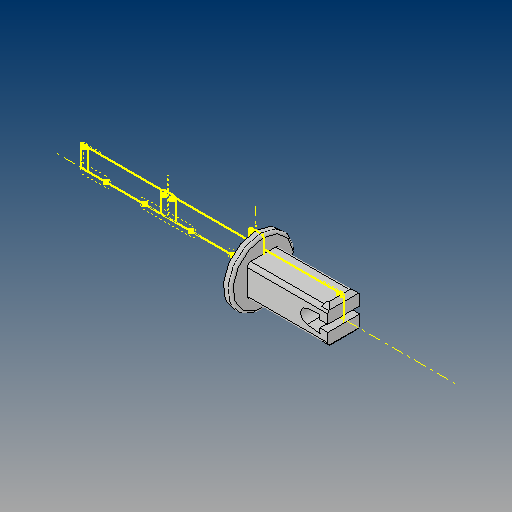
# Autodesk Inventor part: Connector_pin_base
Saved by Autodesk Inventor 2020 (Build 240168000, 168)
## iProperties
Created: 2019-02-01
Part Number: Connector_pin_base
Material: Generic
Document SubType Name: Modeling
Designer: Varga Daniel
Density: 1 g/cm^3
Appearance: Default
Author: Varga Daniel
Autodesk Inventor part; units mm, degrees
ref_plane "YZ Plane" through (0, 0, 0) normal (1, 0, 0) x (0, 1, 0)
ref_plane "XZ Plane" through (0, 0, 0) normal (0, 1, 0) x (-1, 0, 0)
ref_plane "XY Plane" through (0, 0, 0) normal (0, 0, 1) x (1, 0, 0)
derived "Base_part.ipt"
derived "Connector_pin_base.ipt"
sketch "Pin_base_sketch" plane through (0, 0, 0) normal (0, 0, 1) x (1, 0, 0)
  line L0 (0, 0) -> (23.0918, 0) construction
  line L1 (0, 0) -> (0, 6.22) construction
  line L2 (0, 3.75) -> (0.525, 3.75)
  line L3 (0.825, 3.45) -> (0.825, 2.4)
  line L4 (0.825, 2.4) -> (9.225, 2.4)
  line L5 (0, 0) -> (0, 3.75)
  line L6 (0, 0) -> (3.25, 0)
  arc A0 (0.825, 3.45) -> (0.525, 3.75) centre (0.525, 3.45) ccw
  line L7 (0.825, 2.4) -> (0.825, 0.575)
  line L8 (0, 0) -> (-23.0918, 0) construction
  line L9 (9.225, 2.4) -> (9.225, 0.575)
  line L10 (10.025, 2.4) -> (10.025, 2.1865) construction
  line L11 (9.225, 2.4) -> (10.025, 2.4) construction
  line L12 (9.625, 2.4) -> (9.625, 0) construction
  line L13 (10.1291, 2.615) -> (7.4184, 2.615) construction
  line L14 (10.025, 0.575) -> (9.225, 0.575) construction
  line L15 (10.025, 0.575) -> (10.025, 0)
  arc A1 (7.1, 0.575) -> (6.525, 0) centre (7.1, 0) ccw construction
  line L16 (9.225, 0.575) -> (7.1, 0.575) construction
  line L17 (9.225, 0.575) -> (9.225, 0)
  line L18 (0, 0.575) -> (0.825, 0.575) construction
  arc A2 (3.25, 0) -> (2.675, 0.575) centre (2.675, 0) ccw construction
  line L19 (0.825, 0.575) -> (0.825, 0)
  line L20 (0.825, 0.575) -> (2.675, 0.575) construction
  line L21 (0, 0) -> (-3.25, 0)
  line L22 (0, 3.75) -> (-0.525, 3.75)
  line L23 (-0.825, 3.45) -> (-0.825, 2.4)
  arc A3 (-0.525, 3.75) -> (-0.825, 3.45) centre (-0.525, 3.45) ccw
  line L24 (-0.825, 2.4) -> (-0.825, 0.575)
  line L25 (-0.825, 0.575) -> (-0.825, 0)
  line L26 (0, 0.575) -> (-0.825, 0.575) construction
  line L27 (-0.825, 2.4) -> (-9.225, 2.4)
  line L28 (-9.225, 2.4) -> (-9.225, 0)
  line L29 (-10.875, 2.4) -> (-10.875, 0)
  line L30 (-10.5179, 2.55) -> (-9.5821, 2.55)
  line L31 (-10.05, 2.55) -> (-10.05, 0) construction
  line L32 (-9.225, 2.4) -> (-10.875, 2.4) construction
  arc A4 (-10.5179, 2.55) -> (-10.875, 2.4) centre (-10.5179, 2.05) ccw
  arc A5 (-9.225, 2.4) -> (-9.5821, 2.55) centre (-9.5821, 2.05) ccw
  line L33 (-10.875, 2.4) -> (-19.275, 2.4)
  line L34 (-19.275, 2.4) -> (-19.275, 0)
  line L35 (-19.275, 0) -> (-16.575, 0)
  line L36 (-19.275, 2.4) -> (-20.075, 2.4) construction
  line L37 (-20.075, 2.4) -> (-20.075, 2.1865) construction
  line L38 (-20.075, 0) -> (-19.275, 0)
  line L39 (-19.675, 2.4) -> (-19.675, 0) construction
  line L40 (-19.6465, 2.615) -> (-17.4324, 2.615) construction
  line L41 (-0.825, 0.575) -> (-2.675, 0.575) construction
  arc A6 (-2.675, 0.575) -> (-3.25, 0) centre (-2.675, 0) ccw construction
  line L42 (-12.725, 0.575) -> (-7.375, 0.575) construction
  arc A7 (-6.8, 0) -> (-7.375, 0.575) centre (-7.375, 0) ccw construction
  arc A8 (-12.725, 0.575) -> (-13.3, 0) centre (-12.725, 0) ccw construction
  line L43 (-20.075, 0.575) -> (-17.15, 0.575) construction
  arc A9 (-16.575, 0) -> (-17.15, 0.575) centre (-17.15, 0) ccw construction
  line L44 (-16.575, 0) -> (-13.3, 0)
  line L45 (-20.075, 0.575) -> (-20.075, 0)
  line L46 (-13.3, 0) -> (-10.875, 0)
  line L47 (-6.8, 0) -> (-10.875, 0)
  line L48 (-3.25, 0) -> (-6.8, 0)
  line L49 (3.25, 0) -> (6.525, 0)
  line L50 (6.525, 0) -> (10.025, 0)
  arc A10 (-17.15, -0.575) -> (-16.575, 0) centre (-17.15, 0) ccw construction
  line L51 (-20.075, -0.575) -> (-20.075, 0) construction
  line L52 (-20.075, -0.575) -> (-17.15, -0.575) construction
  line L53 (-12.725, -0.575) -> (-7.375, -0.575) construction
  arc A11 (-13.3, 0) -> (-12.725, -0.575) centre (-12.725, 0) ccw construction
  arc A12 (-7.375, -0.575) -> (-6.8, 0) centre (-7.375, 0) ccw construction
  arc A13 (-3.25, 0) -> (-2.675, -0.575) centre (-2.675, 0) ccw construction
  line L54 (-0.825, -0.575) -> (-2.675, -0.575) construction
  line L55 (0, -0.575) -> (-0.825, -0.575) construction
  line L56 (0, -0.575) -> (0.825, -0.575) construction
  line L57 (0.825, -0.575) -> (2.675, -0.575) construction
  arc A14 (2.675, -0.575) -> (3.25, 0) centre (2.675, 0) ccw construction
  arc A15 (6.525, 0) -> (7.1, -0.575) centre (7.1, 0) ccw construction
  line L58 (9.225, -0.575) -> (7.1, -0.575) construction
  line L59 (10.025, -0.575) -> (9.225, -0.575) construction
  line L60 (10.025, -0.575) -> (10.025, 0) construction
  line L61 (-0.025, 0) -> (-0.025, 4.3146) construction
  line L62 (0.025, 0) -> (0.025, 4.3146) construction
  line L63 (-10.075, 0) -> (-10.075, 4.2477) construction
  line L64 (-10.025, 0) -> (-10.025, 4.2339) construction
  arc A16 (-19.275, 2.4) -> (-20.075, 2.1865) centre (-19.6465, 2.1865) ccw
  line L65 (-20.075, 2.1865) -> (-20.075, 0.575)
  arc A17 (10.025, 2.1865) -> (9.225, 2.4) centre (9.5965, 2.1865) ccw
  line L66 (10.025, 2.1865) -> (10.025, 0.575)
sketch "Square_pin_base_sketch" plane through (0, 0, 0) normal (0, 0, 1) x (1, 0, 0)
  line L0 (0, 0) -> (23.0918, 0) construction
  line L1 (0, 3.75) -> (0.525, 3.75)
  line L2 (0.825, 3.45) -> (0.825, 1.825)
  line L3 (0.825, 1.825) -> (9.225, 1.825)
  line L4 (0, 0) -> (0, 3.75)
  line L5 (0, 0) -> (3.25, 0)
  arc A0 (0.825, 3.45) -> (0.525, 3.75) centre (0.525, 3.45) ccw
  line L6 (0.825, 1.825) -> (0.825, 0.575)
  line L7 (0, 0) -> (-23.0918, 0) construction
  line L8 (9.225, 1.825) -> (9.225, 0)
  line L9 (10.025, 1.825) -> (10.025, 1.725) construction
  line L10 (9.225, 1.825) -> (10.025, 1.825) construction
  line L11 (9.625, 2.175) -> (9.625, 0) construction
  line L12 (10.1291, 2.175) -> (7.4184, 2.175) construction
  line L13 (10.025, 0.4) -> (10.025, 0)
  line L14 (0, 0.575) -> (0.825, 0.575)
  arc A1 (3.25, 0) -> (2.675, 0.575) centre (2.675, 0) ccw
  line L15 (0.825, 0.575) -> (0.825, -0.575)
  line L16 (0.825, 0.575) -> (2.675, 0.575)
  line L17 (3.25, 0) -> (6.525, 0)
  line L18 (6.525, 0) -> (10.025, 0)
  line L19 (0, -0.575) -> (0.825, -0.575)
  arc A2 (2.675, -0.575) -> (3.25, 0) centre (2.675, 0) ccw
  line L20 (0.825, -0.575) -> (2.675, -0.575)
  line L21 (10.025, -0.4) -> (10.025, 0) construction
  line L22 (0.025, 0) -> (0.025, 4.3146) construction
  line L23 (10.025, 1.725) -> (10.025, 0)
  line L24 (0, 0.575) -> (0, 0)
  line L25 (0, 0) -> (0, -0.575)
  line L26 (9.625, 2.175) -> (10.025, 1.725)
  arc A3 (9.625, 2.175) -> (9.225, 1.825) centre (9.625, 1.7714) ccw
  line L27 (0, 0) -> (0, 5.1403) construction
  line L28 (10.025, 0.4) -> (9.125, 0.4)
  line L29 (9.125, 0.4) -> (9.125, 0.95)
  line L30 (9.125, 0.95) -> (7.6479, 0.8)
  arc A4 (7.6479, 0.8) -> (6.925, 0) centre (7.7291, 0) ccw
  point P0 (0.825, 0)
  point P1 (-9.225, 0)
  point P2 (-10.875, 0)
  point P3 (-20.075, 0)
  dimension "d237" = 3.65
  dimension "d240" = 0.025
  dimension "d241" = 0.825
  dimension "d242" = 0.3
  dimension "d243" = 7.5
  dimension "d244" = 1.15
  dimension "d245" = 6.5
  dimension "d246" = 8.4
  dimension "d247" = 10
  dimension "d248" = 3.45
  dimension "d249" = 4.35
  dimension "d250" = 0.8
  dimension "d251" = 0.8
  dimension "d252" = 0.9
  dimension "d253" = 1.6
  dimension "d254" = 1.9
  dimension "d255" = 2.3
  constraints: 63 end point, 21 point on line, 13 perpendicular, 10 point on circle, 7 horizontal, 6 tangent, 5 centre point, 4 symmetric about line, 3 collinear, 2 vertical, 1 midpoint, 1 parallel, 3 other
  measures "d237" diameter of L3 L0
  measures "d240" distance between parallel lines of L22 L27
  measures "d241" distance between parallel lines of L4 L2
  measures "d242" radius of A0
  measures "d243" diameter of L1 L7
  measures "d244" distance between parallel lines of L20 L16
  measures "d245" diameter of L5.end L27
  measures "d246" distance between parallel lines of L6 L8
  measures "d247" distance between parallel lines of L23 L22
  measures "d248" diameter of L9.end L0
  measures "d249" diameter of L12 L0
  measures "d250" diameter of L28 L0
  measures "d251" distance between parallel lines of L23 L8
  measures "d252" distance between parallel lines of L23 L29
  measures "d253" diameter of L30.end L0
  measures "d254" diameter of L29.end L0
  measures "d255" distance from line of A4.end L8
revolve "Revolution8" add sketch "Square_pin_base_sketch" angle 360 about axis through (0, 0, 0) along (-1, 0, 0) contours L1 A0 L2 L6 L14 L4 | L14 L15 L5 L4
extrude "Extrusion18" add sketch "Square_pin_base_sketch" along normal mid plane 3.65 contours L16 A1 L5 L15 | L6 L3 L8 L28 L29 L30 A4 L18 L17 A1 L16 | A3 L26 L23 L28 L8
mirror "Mirror1" about plane through (0.825, 0, 0) normal (0, -1, 0) of "Extrusion18"
sketch "Sketch22" plane through (0.825, 0, 0) normal (1, 0, 0) x (0, 0, -1)
  line L0 (1.825, -1.825) -> (-1.825, -1.825) projected
  line L1 (-1.825, -1.825) -> (-1.825, 1.825) projected
  line L2 (-1.825, 1.825) -> (1.825, 1.825) projected
  line L3 (1.825, 1.825) -> (1.825, -1.825) projected
  circle A0 centre (0, 0) radius 3.45 projected
  circle A1 centre (0, 0) radius 3.45 projected
  line L4 (-1.425, 1.825) -> (1.425, 1.825)
  line L5 (1.825, 1.425) -> (1.825, -1.425)
  line L6 (1.425, -1.825) -> (-1.425, -1.825)
  line L7 (-1.825, -1.425) -> (-1.825, 1.425)
  arc A2 (-1.425, 1.825) -> (-1.825, 1.425) centre (-1.425, 1.425) ccw
  arc A3 (1.825, 1.425) -> (1.425, 1.825) centre (1.425, 1.425) ccw
  arc A4 (1.425, -1.825) -> (1.825, -1.425) centre (1.425, -1.425) ccw
  arc A5 (-1.825, -1.425) -> (-1.425, -1.825) centre (-1.425, -1.425) ccw
  line L8 (1.825, -1.825) -> (-1.825, -1.825) projected
  line L9 (-1.825, -1.825) -> (-1.825, 1.825) projected
  line L10 (-1.825, 1.825) -> (1.825, 1.825) projected
  line L11 (1.825, 1.825) -> (1.825, -1.825) projected
  point P0 (-1.825, 1.825)
  point P1 (-1.825, 1.425)
  point P2 (-1.425, 1.825)
  point P3 (-1.425, -1.825)
  point P4 (-1.825, -1.425)
  point P5 (1.825, -1.425)
  point P6 (1.425, -1.825)
  point P7 (1.425, 1.825)
  point P8 (1.825, 1.425)
  dimension "d261" = 0.4
  constraints: 8 end point, 8 point on circle, 8 tangent, 4 centre point, 4 point on line, 3 equal radius, 2 collinear, 2 parallel, 1 horizontal, 1 perpendicular, 1 other
  measures "d261" radius of A2
extrude "Extrusion19" cut sketch "Sketch22" along normal up to surface (8.4 mm away) contours L0 A4 L3 | L0 L1 A5 | A3 L2 L3 | L1 L2 A2
sketch "Sketch21" plane through (10.025, 0.4, 1.825) normal (1, 0, 0) x (0, 0, -1)
  line L0 (0, -1.825) -> (0, 1.025) projected
  arc A0 (0.4, 1.425) -> (0, 1.025) centre (0.4, 1.025) ccw projected
  line L1 (0.4, 1.425) -> (3.25, 1.425) projected
  arc A1 (3.65, 1.025) -> (3.25, 1.425) centre (3.25, 1.025) ccw projected
  line L2 (3.65, 1.025) -> (3.65, -1.825) projected
  arc A2 (3.25, -2.225) -> (3.65, -1.825) centre (3.25, -1.825) ccw projected
  line L3 (3.25, -2.225) -> (0.4, -2.225) projected
  arc A3 (0, -1.825) -> (0.4, -2.225) centre (0.4, -1.825) ccw projected
  circle A4 centre (1.825, -0.4) radius 3.45 projected
  line L4 (3.65, 1.775) -> (0, 1.775) projected
  line L5 (0, 1.325) -> (0, 1.775) projected
  line L6 (3.65, 1.325) -> (0, 1.325) projected
  line L7 (3.65, 1.775) -> (3.65, 1.325) projected
  line L8 (3.65, 1.325) -> (0, 1.325) projected
  line L9 (0, 0) -> (0, 1.325) projected
  line L10 (3.65, 0) -> (0, 0) projected
  line L11 (3.65, 1.325) -> (3.65, 0) projected
  line L12 (3.65, -2.125) -> (0, -2.125) projected
  line L13 (3.65, -2.125) -> (3.65, -0.8) projected
  line L14 (3.65, -0.8) -> (0, -0.8) projected
  line L15 (0, -0.8) -> (0, -2.125) projected
  line L16 (3.65, -2.575) -> (0, -2.575) projected
  line L17 (3.65, -2.575) -> (3.65, -2.125) projected
  line L18 (3.65, -2.125) -> (0, -2.125) projected
  line L19 (0, -2.125) -> (0, -2.575) projected
  line L20 (0.1172, 1.3078) -> (0.5843, 1.775)
  line L21 (3.0657, 1.775) -> (3.5328, 1.3078)
  line L22 (3.5328, -2.1078) -> (3.0657, -2.575)
  line L23 (0.1172, -2.1078) -> (0.5843, -2.575)
  point P0 (3.65, -1.825)
  dimension "d264" = 45
  dimension "d265" = 45
  dimension "d266" = 45
  dimension "d267" = 45
  constraints: 8 end point, 4 point on circle, 4 point on line, 4 tangent
  measures "d264" angle of L20 L5
  measures "d265" angle of L7 L21
  measures "d266" angle of L17 L22
  measures "d267" angle of L19 L23
extrude "Extrusion20" cut sketch "Sketch21" against normal up to surface (0.8 mm away) contours A3 L12 L15 | L12 L23 L16 L19 | L9 L6 A0 | L13 L12 A2 | L12 L17 L16 L22 | L5 L4 L20 L6 | A1 L6 L11 | L6 L21 L4 L7
equation "\"Square_pin_width\" = 3.65"
equation "\"Square_pin_inner_length\" = 8.4"
equation "\"Square_pin_collar_overall_width\" = 4.35"
equation "\"Square_pin_collar_end_width\" = 3.45"
equation "\"Square_pin_gap_end_width\" = 0.8"
equation "\"Square_pin_gap_width_1\" = 1.9"
equation "\"Square_pin_gap_width_2\" = 1.6"
equation "\"Square_pin_gap_length\" = 2.3"
equation "\"Square_pin_collar_height\" = 0.9"
body "Solid8"
